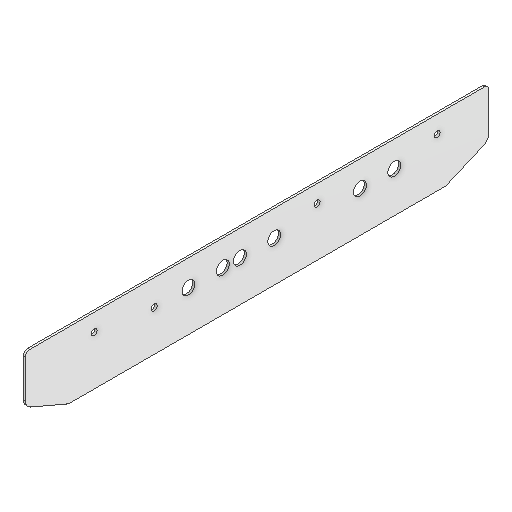
# Autodesk Inventor part: Skirt
Saved by Autodesk Inventor 2025 (Build 290162000, 162)
## iProperties
Created: 2025-01-27
Part Number: Skirt
Material: Acetal Resin, White
Document SubType Name: Modeling
Designer: Averey Ku
Density: 1.425 g/cm^3
Appearance: Smooth - White
Mass: 36.7653 g
Surface Area: 341.862 cm^2
Volume: 25.8002 cm^3
d18: 0.172 in
Author: Averey Ku
Autodesk Inventor part; units mm, degrees
ref_plane "YZ Plane" through (0, 0, 0) normal (1, 0, 0) x (0, 1, 0)
ref_plane "XZ Plane" through (0, 0, 0) normal (0, 1, 0) x (-1, 0, 0)
ref_plane "XY Plane" through (0, 0, 0) normal (0, 0, 1) x (1, 0, 0)
sketch "skirt" plane through (0, 0, 0) normal (0, 0, 1) x (1, 0, 0)
  circle A0 centre (5.0031, 25.9038) radius 4.7625
  line L0 (24.0531, -155.0712) -> (24.0531, 181.4788)
  line L1 (-25.1594, 151.6004) -> (-25.1594, -125.1928)
  circle A1 centre (11.3531, 133.8538) radius 2.1844
  arc A2 (24.0531, 181.4788) -> (20.8781, 184.6538) centre (20.8781, 181.4788) ccw
  line L2 (20.8781, 184.6538) -> (-7.3651, 184.6538)
  line L3 (-24.646, 154.1018) -> (-13.2017, 180.8052)
  arc A3 (-7.3651, 184.6538) -> (-13.2017, 180.8052) centre (-7.3651, 178.3038) ccw
  arc A4 (-24.646, 154.1018) -> (-25.1594, 151.6004) centre (-18.8094, 151.6004) ccw
  line L4 (-24.646, -127.6942) -> (-13.2017, -154.3976)
  line L5 (-7.3651, -158.2462) -> (20.8781, -158.2462)
  arc A5 (20.8781, -158.2462) -> (24.0531, -155.0712) centre (20.8781, -155.0712) ccw
  arc A6 (-25.1594, -125.1928) -> (-24.646, -127.6942) centre (-18.8094, -125.1928) ccw
  circle A7 centre (11.3531, -120.1462) radius 2.1844
  arc A8 (-13.2017, -154.3976) -> (-7.3651, -158.2462) centre (-7.3651, -151.8962) ccw
  circle A9 centre (5.0031, 64.0038) radius 4.7625
  circle A10 centre (5.0031, 38.6038) radius 4.7625
  circle A11 centre (5.0031, 0.5038) radius 4.7625
  circle A12 centre (11.3531, -31.2462) radius 2.1844
  circle A13 centre (5.0031, -62.9962) radius 4.7625
  circle A14 centre (5.0031, -88.3962) radius 4.7625
  circle A15 centre (5.0031, 89.4038) radius 2.1844
  point P0 (-0.9322, -0.2017)
  point P1 (5.0031, 51.3038)
  point P2 (-25.1594, 152.9038)
  point P3 (-25.1594, -126.4962)
  point P4 (5.0031, -12.1962)
  point P5 (5.0031, 13.2038)
  dimension "d0" = 279.4
  dimension "d1" = 49.2125
  dimension "d2" = 3.175
  dimension "d3" = 113.199
  dimension "d4" = 113.199
  dimension "d5" = 6.35
  dimension "d7" = 9.525
  dimension "d13" = 50.8
  dimension "d14" = 38.1
  dimension "d16" = 4.3688
  dimension "d17" = 31.75
  dimension "d18" = 4.3688
  measures "d0" distance of point (-25.159, 152.904) point (-25.159, -126.496)
  measures "d1" distance between parallel lines of L0 L1
  measures "d2" radius of A2
  measures "d3" angle of L2 L3
  measures "d4" angle of L5 L4
  measures "d5" radius of A3
  measures "d7" diameter of A0
  measures "d13" distance from line of A1.centre L2
  measures "d14" distance from line of A7.centre L5
  measures "d16" diameter of A12
  measures "d17" vertical distance of A14.centre A7.centre
  measures "d18" diameter of A15
sketch "Sketch1" plane through (0, 0, 0) normal (1, 0, 0) x (0, 1, 0)
  circle A0 centre (-6.35, -107.95) radius 4.7625
  line L0 (12.7, -288.925) -> (12.7, 47.625)
  line L1 (-36.5125, 17.7466) -> (-36.5125, -259.0466)
  circle A1 centre (0, 0) radius 2.1844
  arc A2 (12.7, 47.625) -> (9.525, 50.8) centre (9.525, 47.625) ccw
  line L2 (9.525, 50.8) -> (-18.7182, 50.8)
  line L3 (-35.9991, 20.248) -> (-24.5548, 46.9514)
  arc A3 (-18.7182, 50.8) -> (-24.5548, 46.9514) centre (-18.7182, 44.45) ccw
  arc A4 (-35.9991, 20.248) -> (-36.5125, 17.7466) centre (-30.1625, 17.7466) ccw
  line L4 (-35.9991, -261.548) -> (-24.5548, -288.2514)
  line L5 (-18.7182, -292.1) -> (9.525, -292.1)
  arc A5 (9.525, -292.1) -> (12.7, -288.925) centre (9.525, -288.925) ccw
  arc A6 (-36.5125, -259.0466) -> (-35.9991, -261.548) centre (-30.1625, -259.0466) ccw
  circle A7 centre (0, -254) radius 2.1844
  arc A8 (-24.5548, -288.2514) -> (-18.7182, -292.1) centre (-18.7182, -285.75) ccw
  circle A9 centre (-6.35, -69.85) radius 4.7625
  circle A10 centre (-6.35, -95.25) radius 4.7625
  circle A11 centre (-6.35, -133.35) radius 4.7625
  circle A12 centre (0, -165.1) radius 2.1844
  circle A13 centre (-6.35, -196.85) radius 4.7625
  circle A14 centre (-6.35, -222.25) radius 4.7625
  circle A15 centre (-6.35, -44.45) radius 2.1844
  constraints: 1 other
extrude "Extrusion1" add sketch "Sketch1" along normal blind 1.5875
body "Solid1"
